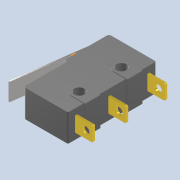
# Autodesk Inventor part: Omron微動(精確)
Saved by Autodesk Inventor 2020.2 (Build 242310000, 310)
## iProperties
Created: 2020-09-06
Part Number: Omron微動(精確)
Material: 一般
Document SubType Name: Modeling
Designer: 108033238朱軒毅
Density: 1 g/cm^3
Appearance: 預設
Author: 108033238朱軒毅
Autodesk Inventor part; units mm, degrees
ref_plane "YZ Plane" through (0, 0, 0) normal (1, 0, 0) x (0, 1, 0)
ref_plane "XZ Plane" through (0, 0, 0) normal (0, 1, 0) x (-1, 0, 0)
ref_plane "XY Plane" through (0, 0, 0) normal (0, 0, 1) x (1, 0, 0)
sketch "草圖1" plane through (0, 0, 0) normal (0, 1, 0) x (-1, 0, 0)
  line L0 (5.325, 9.95) -> (-5.325, 9.95)
  line L1 (-5.325, 9.95) -> (-5.325, -9.95)
  line L2 (-5.325, -9.95) -> (5.325, -9.95)
  line L3 (5.325, -9.95) -> (5.325, 9.95)
  line L4 (5.325, 9.95) -> (-5.325, -9.95) construction
  line L5 (-5.325, 9.95) -> (5.325, -9.95) construction
  point P0 (0, 0)
  dimension "d0" = 10.65
  dimension "d1" = 19.9
  constraints: 12 end point, 2 midpoint, 2 parallel, 1 horizontal, 1 perpendicular
  measures "d0" distance of L2.end L1.end
  measures "d1" distance of L1.end L0.end
extrude "擠出1" add sketch "草圖1" along normal mid plane 6.16
sketch "草圖2" plane through (0, 3.08, 0) normal (0, 1, 0) x (1, 0, 0)
  line L0 (-5.325, 9.95) -> (-5.325, -9.95) projected
  line L1 (-5.325, -9.95) -> (5.325, -9.95) projected
  line L2 (5.325, -9.95) -> (5.325, 9.95) projected
  line L3 (-5.325, 0) -> (-4.675, 0)
  line L4 (-4.675, 0) -> (-4.675, -9.95)
  point P0 (0, 0)
  dimension "d4" = 10
  constraints: 4 end point, 1 horizontal, 1 horizontal alignment, 1 midpoint, 1 perpendicular, 1 point on line
  measures "d4" distance between parallel lines of L2 L4
extrude "擠出2" cut sketch "草圖2" against normal through all
sketch "草圖3" plane through (0, 0, 0) normal (0, 1, 0) x (-1, 0, 0)
  line L0 (4.675, 9.95) -> (4.675, 0) projected
  line L1 (4.675, 0) -> (5.325, 0) projected
  line L2 (5.325, 0) -> (5.325, -9.95) projected
  line L3 (5.325, -9.95) -> (-5.325, -9.95) projected
  line L4 (-5.325, -9.95) -> (-5.325, 9.95) projected
  line L5 (-5.325, 9.95) -> (4.675, 9.95) projected
  line L6 (-5.725, 6.45) -> (-2.675, 6.45)
  arc A0 (-2.675, 3.05) -> (-2.675, 6.45) centre (-2.675, 4.75) ccw
  line L7 (-2.675, 3.05) -> (-5.725, 3.05)
  line L8 (-5.725, 3.05) -> (-5.725, 6.45)
  line L9 (-5.725, -3.05) -> (-2.675, -3.05)
  arc A1 (-2.675, -6.45) -> (-2.675, -3.05) centre (-2.675, -4.75) ccw
  line L10 (-2.675, -6.45) -> (-5.725, -6.45)
  line L11 (-5.725, -6.45) -> (-5.725, -3.05)
  point P0 (0, 0)
  point P1 (-0.975, 4.75)
  point P2 (-0.975, -4.75)
  dimension "d9" = 0.4
  dimension "d10" = 4.75
  dimension "d15" = 9.5
  dimension "d17" = 3.4
  dimension "d18" = 3.5
  constraints: 12 end point, 6 point on circle, 5 perpendicular, 4 tangent, 2 centre point, 2 horizontal alignment, 2 point on line, 2 vertical alignment, 1 equal radius, 1 horizontal
  measures "d9" distance between parallel lines of L4 L11
  measures "d10" distance from line of L11 point (-0.975, -4.75)
  measures "d15" distance of A1.centre A0.centre
  measures "d17" distance between parallel lines of L7 L6
  measures "d18" distance between parallel lines of L5 L6
extrude "擠出3" add sketch "草圖3" along normal mid plane 6.48 contours L6 A0 L7 L4 | L4 L7 L8 L6 | L9 A1 L10 L4 | L4 L10 L11 L9
sketch "草圖4" plane through (0, 3.24, 0) normal (0, 1, 0) x (1, 0, 0)
  arc A0 (2.675, -3.05) -> (2.675, -6.45) centre (2.675, -4.75) ccw projected
  circle A1 centre (2.675, -4.75) radius 1.15
  line L0 (5.725, 3.05) -> (5.725, 6.45) projected
  line L1 (5.725, 6.45) -> (2.675, 6.45) projected
  arc A2 (2.675, 6.45) -> (2.675, 3.05) centre (2.675, 4.75) ccw projected
  line L2 (2.675, 3.05) -> (5.725, 3.05) projected
  circle A3 centre (2.675, 4.75) radius 1.15
  point P0 (0, 0)
  dimension "d19" = 2.3
  constraints: 2 centre point, 2 coincident, 1 equal radius
  measures "d19" diameter of A1
extrude "擠出4" cut sketch "草圖4" against normal through all contours A1 | A3
sketch "草圖5" plane through (0, 0, 0) normal (0, 1, 0) x (-1, 0, 0)
  circle A0 centre (-2.675, -4.75) radius 1.15 projected
  circle A1 centre (-2.675, 4.75) radius 1.15 projected
  line L0 (4.675, 9.95) -> (4.675, 0) projected
  line L1 (4.675, 0) -> (5.325, 0) projected
  line L2 (5.325, 0) -> (5.325, -9.95) projected
  line L3 (5.325, -9.95) -> (-5.325, -9.95) projected
  line L4 (-5.325, -9.95) -> (-5.325, -6.45) projected
  line L5 (-5.325, -6.45) -> (-5.725, -6.45) projected
  line L6 (-5.725, -6.45) -> (-5.725, -3.05) projected
  line L7 (-5.725, -3.05) -> (-5.325, -3.05) projected
  line L8 (-5.325, -3.05) -> (-5.325, 3.05) projected
  line L9 (-5.325, 3.05) -> (-5.725, 3.05) projected
  line L10 (-5.725, 3.05) -> (-5.725, 6.45) projected
  line L11 (-5.725, 6.45) -> (-5.325, 6.45) projected
  line L12 (-5.325, 6.45) -> (-5.325, 9.95) projected
  line L13 (-5.325, 9.95) -> (4.675, 9.95) projected
  line L14 (-5.325, 8.35) -> (-9.325, 8.35)
  line L15 (-9.325, 8.35) -> (-9.325, 7.85)
  line L16 (-9.325, 7.85) -> (-5.325, 7.85)
  line L17 (-5.325, 7.85) -> (-5.325, 8.35)
  line L18 (-5.325, 0.85) -> (-9.325, 0.85)
  line L19 (-9.325, 0.85) -> (-9.325, 0.35)
  line L20 (-9.325, 0.35) -> (-5.325, 0.35)
  line L21 (-5.325, 0.35) -> (-5.325, 0.85)
  line L22 (-5.325, -7.95) -> (-9.325, -7.95)
  line L23 (-9.325, -7.95) -> (-9.325, -8.45)
  line L24 (-9.325, -8.45) -> (-5.325, -8.45)
  line L25 (-5.325, -8.45) -> (-5.325, -7.95)
  point P0 (0, 0)
  dimension "d22" = 0.5
  dimension "d23" = 1.5
  dimension "d24" = 8.3
  dimension "d25" = 7
  dimension "d26" = 3.6
  constraints: 24 end point, 6 parallel, 5 point on line, 3 horizontal, 3 perpendicular, 2 collinear
  measures "d22" distance of L14.end L15.end
  measures "d23" distance between parallel lines of L3 L24
  measures "d24" distance between parallel lines of L20 L22
  measures "d25" distance between parallel lines of L16 L18
  measures "d26" distance between parallel lines of L10 L15
extrude "擠出5" add sketch "草圖5" along normal mid plane 3.33 contours L12 L16 L15 L14 | L24 L23 L22 L4 | L8 L20 L19 L18
sketch "草圖6" plane through (5.325, 1.665, 8.35) normal (0, 0, 1) x (1, 0, 0)
  line L0 (4, -3.33) -> (4, 0) projected
  circle A0 centre (2.45, -1.665) radius 0.8
  point P0 (-5.325, -1.665)
  point P1 (4, -1.665)
  point P2 (3.25, -1.665)
  dimension "d29" = 1.6
  dimension "d30" = 0.75
  constraints: 3 horizontal alignment, 1 midpoint, 2 other
  measures "d30" distance of point (4, -1.665) point (3.25, -1.665)
extrude "擠出6" cut sketch "草圖6" against normal through all
sketch "草圖7" plane through (0, 0, 0) normal (0, 1, 0) x (-1, 0, 0)
  line L0 (-9.325, -8.45) -> (-9.325, -7.95) projected
  line L1 (-9.325, -7.95) -> (-8.575, -7.95) projected
  line L2 (-8.575, -7.95) -> (-8.575, -8.45) projected
  line L3 (-8.575, -8.45) -> (-9.325, -8.45) projected
  line L4 (-9.325, 0.35) -> (-9.325, 0.85) projected
  line L5 (-9.325, 0.85) -> (-8.575, 0.85) projected
  line L6 (-8.575, 0.85) -> (-8.575, 0.35) projected
  line L7 (-8.575, 0.35) -> (-9.325, 0.35) projected
  line L8 (-9.325, 7.85) -> (-9.325, 8.35) projected
  line L9 (-9.325, 8.35) -> (-8.575, 8.35) projected
  line L10 (-8.575, 8.35) -> (-8.575, 7.85) projected
  line L11 (-8.575, 7.85) -> (-9.325, 7.85) projected
  circle A0 centre (-2.675, -4.75) radius 1.15 projected
  circle A1 centre (-2.675, 4.75) radius 1.15 projected
  line L12 (4.675, 9.95) -> (4.675, 0) projected
  line L13 (4.675, 0) -> (5.325, 0) projected
  line L14 (5.325, 0) -> (5.325, -9.95) projected
  line L15 (5.325, -9.95) -> (-5.325, -9.95) projected
  line L16 (-5.325, -9.95) -> (-5.325, -8.45) projected
  line L17 (-5.325, -8.45) -> (-6.975, -8.45) projected
  line L18 (-6.975, -8.45) -> (-6.975, -7.95) projected
  line L19 (-6.975, -7.95) -> (-5.325, -7.95) projected
  line L20 (-5.325, -7.95) -> (-5.325, -6.45) projected
  line L21 (-5.325, -6.45) -> (-5.725, -6.45) projected
  line L22 (-5.725, -6.45) -> (-5.725, -3.05) projected
  line L23 (-5.725, -3.05) -> (-5.325, -3.05) projected
  line L24 (-5.325, -3.05) -> (-5.325, 0.35) projected
  line L25 (-5.325, 0.35) -> (-6.975, 0.35) projected
  line L26 (-6.975, 0.35) -> (-6.975, 0.85) projected
  line L27 (-6.975, 0.85) -> (-5.325, 0.85) projected
  line L28 (-5.325, 0.85) -> (-5.325, 3.05) projected
  line L29 (-5.325, 3.05) -> (-5.725, 3.05) projected
  line L30 (-5.725, 3.05) -> (-5.725, 6.45) projected
  line L31 (-5.725, 6.45) -> (-5.325, 6.45) projected
  line L32 (-5.325, 6.45) -> (-5.325, 7.85) projected
  line L33 (-5.325, 7.85) -> (-6.975, 7.85) projected
  line L34 (-6.975, 7.85) -> (-6.975, 8.35) projected
  line L35 (-6.975, 8.35) -> (-5.325, 8.35) projected
  line L36 (-5.325, 8.35) -> (-5.325, 9.95) projected
  line L37 (-5.325, 9.95) -> (4.675, 9.95) projected
  line L38 (5.325, -1.75) -> (5.375, -1.75)
  arc A2 (5.375, -4.15) -> (5.375, -1.75) centre (5.375, -2.95) ccw
  line L39 (5.375, -4.15) -> (5.325, -4.15)
  point P0 (0, 0)
  dimension "d33" = 1.2
  dimension "d34" = 0.05
  dimension "d35" = 7
  constraints: 4 end point, 2 perpendicular, 2 point on circle, 2 point on line, 2 tangent, 1 centre point
  measures "d33" radius of A2
  measures "d34" distance from line of L14 A2.centre
  measures "d35" distance from line of L15 A2.centre
extrude "擠出7" add sketch "草圖7" along normal mid plane 4.2 contours L38 A2 L39 L14
sketch "草圖8" plane through (0, 0, 0) normal (0, 1, 0) x (-1, 0, 0)
  line L0 (-9.325, -8.45) -> (-9.325, -7.95) projected
  line L1 (-9.325, -7.95) -> (-8.575, -7.95) projected
  line L2 (-8.575, -7.95) -> (-8.575, -8.45) projected
  line L3 (-8.575, -8.45) -> (-9.325, -8.45) projected
  line L4 (-9.325, 0.35) -> (-9.325, 0.85) projected
  line L5 (-9.325, 0.85) -> (-8.575, 0.85) projected
  line L6 (-8.575, 0.85) -> (-8.575, 0.35) projected
  line L7 (-8.575, 0.35) -> (-9.325, 0.35) projected
  line L8 (-9.325, 7.85) -> (-9.325, 8.35) projected
  line L9 (-9.325, 8.35) -> (-8.575, 8.35) projected
  line L10 (-8.575, 8.35) -> (-8.575, 7.85) projected
  line L11 (-8.575, 7.85) -> (-9.325, 7.85) projected
  circle A0 centre (-2.675, -4.75) radius 1.15 projected
  circle A1 centre (-2.675, 4.75) radius 1.15 projected
  line L12 (4.675, 9.95) -> (4.675, 0) projected
  line L13 (4.675, 0) -> (5.325, 0) projected
  line L14 (5.325, 0) -> (5.325, -1.75) projected
  line L15 (5.325, -4.15) -> (5.325, -9.95) projected
  line L16 (5.325, -9.95) -> (-5.325, -9.95) projected
  line L17 (-5.325, -9.95) -> (-5.325, -8.45) projected
  line L18 (-5.325, -8.45) -> (-6.975, -8.45) projected
  line L19 (-6.975, -8.45) -> (-6.975, -7.95) projected
  line L20 (-6.975, -7.95) -> (-5.325, -7.95) projected
  line L21 (-5.325, -7.95) -> (-5.325, -6.45) projected
  line L22 (-5.325, -6.45) -> (-5.725, -6.45) projected
  line L23 (-5.725, -6.45) -> (-5.725, -3.05) projected
  line L24 (-5.725, -3.05) -> (-5.325, -3.05) projected
  line L25 (-5.325, -3.05) -> (-5.325, 0.35) projected
  line L26 (-5.325, 0.35) -> (-6.975, 0.35) projected
  line L27 (-6.975, 0.35) -> (-6.975, 0.85) projected
  line L28 (-6.975, 0.85) -> (-5.325, 0.85) projected
  line L29 (-5.325, 0.85) -> (-5.325, 3.05) projected
  line L30 (-5.325, 3.05) -> (-5.725, 3.05) projected
  line L31 (-5.725, 3.05) -> (-5.725, 6.45) projected
  line L32 (-5.725, 6.45) -> (-5.325, 6.45) projected
  line L33 (-5.325, 6.45) -> (-5.325, 7.85) projected
  line L34 (-5.325, 7.85) -> (-6.975, 7.85) projected
  line L35 (-6.975, 7.85) -> (-6.975, 8.35) projected
  line L36 (-6.975, 8.35) -> (-5.325, 8.35) projected
  line L37 (-5.325, 8.35) -> (-5.325, 9.95) projected
  line L38 (-5.325, 9.95) -> (4.675, 9.95) projected
  line L39 (5.325, -6.95) -> (6.325, -6.95)
  line L40 (6.325, -6.95) -> (8.6351, 9.408)
  line L41 (8.6351, 9.408) -> (8.338, 9.45)
  line L42 (8.338, 9.45) -> (6.0644, -6.65)
  line L43 (6.0644, -6.65) -> (5.325, -6.65)
  line L44 (5.325, -1.75) -> (5.375, -1.75) projected
  arc A2 (5.375, -4.15) -> (5.375, -1.75) centre (5.375, -2.95) ccw projected
  line L45 (5.375, -4.15) -> (5.325, -4.15) projected
  arc A3 (5.375, -4.15) -> (5.375, -1.75) centre (5.375, -2.95) ccw projected
  point P0 (0, 0)
  dimension "d38" = 0.3
  dimension "d39" = 0.3
  dimension "d40" = 3
  dimension "d41" = 1
  dimension "d42" = 0.5
  constraints: 10 end point, 2 parallel, 2 perpendicular, 2 point on line, 1 tangent
  measures "d38" distance between parallel lines of L42 L40
  measures "d39" distance between parallel lines of L43 L39
  measures "d40" distance between parallel lines of L16 L39
  measures "d41" distance from line of L15 L39.end
  measures "d42" vertical distance of L12.start L41.end
extrude "擠出8" add sketch "草圖8" along normal mid plane 4 contours L42 L41 L40 L39 L15 L43
fillet "圓角1" radius 0.2 2 edges at (-6.0644, 0, -6.65) (-6.325, 0, -6.95)
fillet "圓角2" radius 0.5 4 edges at (-5.325, 0, 0) (-4.675, 0, 0) (-4.675, 0, 9.95) (-5.325, 0, -9.95)
fillet "圓角2" radius 0.25 2 edges at (5.325, 0, 9.95) (5.325, 0, -9.95)
fillet "圓角3" radius 0.25 6 edges at (9.325, 1.665, 0.6) (9.325, -1.665, 0.6) (9.325, 1.665, -8.2) (9.325, -1.665, -8.2) (9.325, 1.665, 8.1) (9.325, -1.665, 8.1)
equation "\"d39\" = d38"
